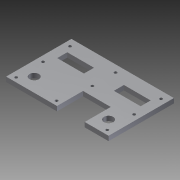
# Autodesk Inventor part: carro x lado polea pieza4 tapa
Saved by Autodesk Inventor 2012 (Build 160160000, 160)
## iProperties
Created: 2014-12-17
Part Number: carro x lado polea pieza4 tapa
Material: Default
Document SubType Name: Modeling
Designer: PRINCIPAL
Density: 1 g/cm^3
Author: PRINCIPAL
Autodesk Inventor part; units mm, degrees
ref_plane "YZ Plane" through (0, 0, 0) normal (1, 0, 0) x (0, 1, 0)
ref_plane "XZ Plane" through (0, 0, 0) normal (0, 1, 0) x (-1, 0, 0)
ref_plane "XY Plane" through (0, 0, 0) normal (0, 0, 1) x (1, 0, 0)
sketch "Boceto1" plane through (0, 0, 0) normal (0, 0, 1) x (1, 0, 0)
  arc A0 (-18.1173, 21.3488) -> (-19.6673, 19.7988) centre (-18.1173, 19.7988) ccw
  arc A1 (-19.6673, 19.7988) -> (-18.1173, 18.2488) centre (-18.1173, 19.7988) ccw
  arc A2 (-18.1173, 18.2488) -> (-16.5673, 19.7988) centre (-18.1173, 19.7988) ccw
  arc A3 (-16.5673, 19.7988) -> (-18.1173, 21.3488) centre (-18.1173, 19.7988) ccw
  arc A4 (-18.1173, -7.6512) -> (-19.6673, -9.2012) centre (-18.1173, -9.2012) ccw
  arc A5 (-19.6673, -9.2012) -> (-18.1173, -10.7512) centre (-18.1173, -9.2012) ccw
  arc A6 (-18.1173, -10.7512) -> (-16.5673, -9.2012) centre (-18.1173, -9.2012) ccw
  arc A7 (-16.5673, -9.2012) -> (-18.1173, -7.6512) centre (-18.1173, -9.2012) ccw
  arc A8 (-18.1173, -36.6512) -> (-19.6673, -38.2012) centre (-18.1173, -38.2012) ccw
  arc A9 (-19.6673, -38.2012) -> (-18.1173, -39.7512) centre (-18.1173, -38.2012) ccw
  arc A10 (-18.1173, -39.7512) -> (-16.5673, -38.2012) centre (-18.1173, -38.2012) ccw
  arc A11 (-16.5673, -38.2012) -> (-18.1173, -36.6512) centre (-18.1173, -38.2012) ccw
  arc A12 (-67.1173, 21.3488) -> (-68.6673, 19.7988) centre (-67.1173, 19.7988) ccw
  arc A13 (-68.6673, 19.7988) -> (-67.1173, 18.2488) centre (-67.1173, 19.7988) ccw
  arc A14 (-67.1173, 18.2488) -> (-65.5673, 19.7988) centre (-67.1173, 19.7988) ccw
  arc A15 (-65.5673, 19.7988) -> (-67.1173, 21.3488) centre (-67.1173, 19.7988) ccw
  arc A16 (-67.1173, -3.6326) -> (-68.6673, -5.1826) centre (-67.1173, -5.1826) ccw
  arc A17 (-68.6673, -5.1826) -> (-67.1173, -6.7326) centre (-67.1173, -5.1826) ccw
  arc A18 (-67.1173, -6.7326) -> (-65.5673, -5.1826) centre (-67.1173, -5.1826) ccw
  arc A19 (-65.5673, -5.1826) -> (-67.1173, -3.6326) centre (-67.1173, -5.1826) ccw
  arc A20 (-72.6173, -36.6512) -> (-74.1673, -38.2012) centre (-72.6173, -38.2012) ccw
  arc A21 (-74.1673, -38.2012) -> (-72.6173, -39.7512) centre (-72.6173, -38.2012) ccw
  arc A22 (-72.6173, -39.7512) -> (-71.0673, -38.2012) centre (-72.6173, -38.2012) ccw
  arc A23 (-71.0673, -38.2012) -> (-72.6173, -36.6512) centre (-72.6173, -38.2012) ccw
  arc A24 (-116.1173, 21.3488) -> (-117.6673, 19.7988) centre (-116.1173, 19.7988) ccw
  arc A25 (-117.6673, 19.7988) -> (-116.1173, 18.2488) centre (-116.1173, 19.7988) ccw
  arc A26 (-116.1173, 18.2488) -> (-114.5673, 19.7988) centre (-116.1173, 19.7988) ccw
  arc A27 (-114.5673, 19.7988) -> (-116.1173, 21.3488) centre (-116.1173, 19.7988) ccw
  arc A28 (-116.1173, -7.6512) -> (-117.6673, -9.2012) centre (-116.1173, -9.2012) ccw
  arc A29 (-117.6673, -9.2012) -> (-116.1173, -10.7512) centre (-116.1173, -9.2012) ccw
  arc A30 (-116.1173, -10.7512) -> (-114.5673, -9.2012) centre (-116.1173, -9.2012) ccw
  arc A31 (-114.5673, -9.2012) -> (-116.1173, -7.6512) centre (-116.1173, -9.2012) ccw
  arc A32 (-116.1173, -36.6512) -> (-117.6673, -38.2012) centre (-116.1173, -38.2012) ccw
  arc A33 (-117.6673, -38.2012) -> (-116.1173, -39.7512) centre (-116.1173, -38.2012) ccw
  arc A34 (-116.1173, -39.7512) -> (-114.5673, -38.2012) centre (-116.1173, -38.2012) ccw
  arc A35 (-114.5673, -38.2012) -> (-116.1173, -36.6512) centre (-116.1173, -38.2012) ccw
  arc A36 (-107.1173, -22.7512) -> (-112.0673, -27.7012) centre (-107.1173, -27.7012) ccw
  arc A37 (-112.0673, -27.7012) -> (-107.1173, -32.6512) centre (-107.1173, -27.7012) ccw
  arc A38 (-107.1173, -32.6512) -> (-102.1673, -27.7012) centre (-107.1173, -27.7012) ccw
  arc A39 (-102.1673, -27.7012) -> (-107.1173, -22.7512) centre (-107.1173, -27.7012) ccw
  arc A40 (-27.1173, -22.7512) -> (-32.0673, -27.7012) centre (-27.1173, -27.7012) ccw
  arc A41 (-32.0673, -27.7012) -> (-27.1173, -32.6512) centre (-27.1173, -27.7012) ccw
  arc A42 (-27.1173, -32.6512) -> (-22.1673, -27.7012) centre (-27.1173, -27.7012) ccw
  arc A43 (-22.1673, -27.7012) -> (-27.1173, -22.7512) centre (-27.1173, -27.7012) ccw
  line L0 (-83.2173, 1.8988) -> (-83.2173, 12.6988)
  line L1 (-83.2173, 12.6988) -> (-112.0173, 12.6988)
  line L2 (-112.0173, 12.6988) -> (-112.0173, 1.8988)
  line L3 (-112.0173, 1.8988) -> (-83.2173, 1.8988)
  line L4 (-22.2173, 1.8988) -> (-22.2173, 12.6988)
  line L5 (-22.2173, 12.6988) -> (-51.0173, 12.6988)
  line L6 (-51.0173, 12.6988) -> (-51.0173, 1.8988)
  line L7 (-51.0173, 1.8988) -> (-22.2173, 1.8988)
  line L8 (-67.4673, -14.8512) -> (-37.6673, -14.8512)
  line L9 (-37.6673, -14.8512) -> (-37.6673, -42.8512)
  line L10 (-37.6673, -42.8512) -> (-11.9673, -42.8512)
  line L11 (-11.9673, -42.8512) -> (-11.9673, 27.4488)
  line L12 (-11.9673, 27.4488) -> (-122.2673, 27.4488)
  line L13 (-122.2673, 27.4488) -> (-122.2673, -42.8512)
  line L14 (-122.2673, -42.8512) -> (-67.4673, -42.8512)
  line L15 (-67.4673, -42.8512) -> (-67.4673, -14.8512)
  point P0 (0, 0)
  constraints: 88 point on circle, 44 centre point, 32 end point
extrude "Extrusión1" add sketch "Boceto1" along normal blind 5
